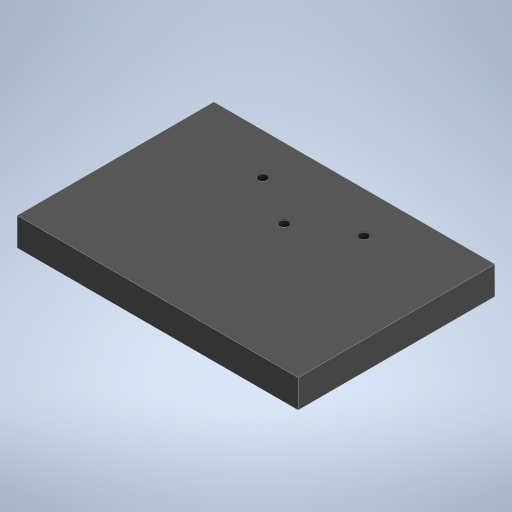
# Autodesk Inventor part: toe_sole_front
Saved by Autodesk Inventor 2024.1 (Build 281209000, 209)
## iProperties
Created: 2024-02-12
Part Number: toe_sole_front
Material: 一般
Document SubType Name: モデリング
Designer: hibik
Density: 1 g/cm^3
Appearance: 既定
Author: hibik
Autodesk Inventor part; units mm, degrees
ref_plane "YZ Plane" through (0, 0, 0) normal (1, 0, 0) x (0, 1, 0)
ref_plane "XZ Plane" through (0, 0, 0) normal (0, 1, 0) x (-1, 0, 0)
ref_plane "XY Plane" through (0, 0, 0) normal (0, 0, 1) x (1, 0, 0)
sketch "スケッチ1" plane through (0, 0, 0) normal (0, 1, 0) x (-1, 0, 0)
  line L0 (26, 0) -> (0, 0)
  line L1 (0, 0) -> (0, -15)
  line L2 (0, -15) -> (26, -15)
  line L3 (26, -15) -> (26, 0)
  line L4 (36.4849, 5.9511) -> (26, -20)
  line L5 (26, -20) -> (0, -20)
  line L6 (0, -20) -> (-10.4849, 5.9511)
  arc A0 (36.4849, 5.9511) -> (-10.4849, 5.9511) centre (13, -20) ccw
  line L7 (0, 0) -> (26, -15)
  line L8 (0, -15) -> (26, 0)
  line L9 (4, -2.3077) -> (22, -2.3077)
  line L10 (22, -2.3077) -> (22, -12.6923)
  line L11 (22, -12.6923) -> (4, -12.6923)
  line L12 (4, -12.6923) -> (4, -2.3077)
  circle A1 centre (4, -2.3077) radius 0.8
  circle A2 centre (4, -12.6923) radius 0.8
  circle A3 centre (22, -2.3077) radius 0.8
  circle A4 centre (22, -12.6923) radius 0.8
  circle A5 centre (13, -7.5) radius 0.8
  line L13 (38, 15) -> (-12, 15)
  line L14 (-12, 15) -> (-12, -20)
  line L15 (-12, -20) -> (38, -20)
  line L16 (38, -20) -> (38, 15)
  point P0 (22.6929, -13.0921)
  point P1 (21.2, -12.6923)
  point P2 (13, 15)
  point P3 (13, -7.5)
  point P4 (13, 15)
  point P5 (0, -20)
  dimension "d0" = 26
  dimension "d1" = 15
  dimension "d4" = 22
  dimension "d5" = 22
  dimension "d6" = 5
  dimension "d7" = 35
  dimension "d23" = 4
  dimension "d24" = 1.6
  dimension "d25" = 1.6
  dimension "d26" = 1.6
  dimension "d27" = 1.6
  dimension "d32" = 1.6
  dimension "d54" = 50
  dimension "d55" = 35
  constraints: 34 end point, 6 centre point, 6 coincident, 6 parallel, 5 point on line, 4 horizontal, 4 midpoint, 3 perpendicular, 2 point on circle, 1 collinear, 1 vertical alignment
  measures "d0" distance of L0.start L0.end
  measures "d1" distance of L2.end L0.start
  measures "d4" angle of L3 L4
  measures "d5" angle of L6 L1
  measures "d6" distance between parallel lines of L5 L2
  measures "d7" radius of A0
  measures "d23" distance between parallel lines of L1 L12
  measures "d24" diameter of A1
  measures "d25" diameter of A2
  measures "d26" diameter of A3
  measures "d27" diameter of A4
  measures "d32" diameter of A5
  measures "d54" distance of L13.start L13.end
  measures "d55" distance of L13.end L14.end
extrude "押し出し1" add sketch "スケッチ1" along normal blind 4 contours L8 A3 L9 A1 L7 L0 | L3 L7 A4 L10 A3 L8 | L7 A1 L12 A2 L8 L1 | L2 L8 A2 L11 A4 L7 | A3 L10 L8 | L8 L9 A3 | A1 L9 L7 | L7 L12 A1 | L10 A3 L8 | L8 A3 L9 | A3 L8 A5 L7 A1 L9 | L9 A1 L7 | L7 A1 L12 | A1 L7 A5 L8 A2 L12 | L11 A2 L8 A5 L7 A4 | A3 L10 A4 L7 A5 L8 | A0 L13 L16 L15 L4 | L4 L5 L6 A0 | A0 L6 L15 L14 L13
sketch "スケッチ5" plane through (0, 0, 0) normal (0, -1, 0) x (1, 0, 0)
  line L0 (12, -20) -> (-38, -20) projected
  line L1 (12, 15) -> (12, -20) projected
  line L2 (-38, 15) -> (12, 15) projected
  line L3 (-38, -20) -> (-38, 15) projected
  circle A0 centre (-13, -7.5) radius 0.8 projected
  circle A1 centre (-4, -12.6923) radius 0.8 projected
  circle A2 centre (-22, -12.6923) radius 0.8 projected
  circle A3 centre (-13, -7.5) radius 2.5
  circle A4 centre (-4, -12.6923) radius 2.5
  circle A5 centre (-22, -12.6923) radius 2.5
  line L4 (10, 12.5) -> (2, 12.5)
  line L5 (2, 12.5) -> (2, -17.5)
  line L6 (2, -17.5) -> (10, -17.5)
  line L7 (10, -17.5) -> (10, 12.5)
  line L8 (-28, 12.5) -> (-36, 12.5)
  line L9 (-36, 12.5) -> (-36, -17.5)
  line L10 (-36, -17.5) -> (-28, -17.5)
  line L11 (-28, -17.5) -> (-28, 12.5)
  point P0 (0, 0)
  point P1 (10, -2.5)
  point P2 (12, -2.5)
  point P3 (-28, -2.5)
  dimension "d56" = 5
  dimension "d57" = 5
  dimension "d58" = 5
  dimension "d61" = 8
  dimension "d62" = 30
  dimension "d63" = 2
  dimension "d64" = 2
  constraints: 16 end point, 4 parallel, 3 centre point, 3 coincident, 3 midpoint, 2 equal length, 2 horizontal, 2 horizontal alignment, 2 perpendicular
  measures "d56" diameter of A3
  measures "d57" diameter of A4
  measures "d58" diameter of A5
  measures "d61" distance of L6.end L5.end
  measures "d62" distance of L5.end L4.end
  measures "d63" distance between parallel lines of L1 L7
  measures "d64" distance between parallel lines of L3 L9
extrude "押し出し5" add sketch "スケッチ5" along normal blind 1 contours L0 L3 L2 L1
fillet "フィレット3" radius 1 8 edges at (6, -1, 12.5) (10, -1, -2.5) (6, -1, -17.5) (2, -1, -2.5) (-28, -1, -2.5) (-32, -1, -17.5) (-36, -1, -2.5) (-32, -1, 12.5)
equation "\"d5\" = d4"
equation "\"BendRadius\" = Thickness"
equation "\"BendReliefWidth\" = Thickness"
equation "\"BendReliefDepth\" = 0.5 * Thickness"
equation "\"CornerReliefSize\" = 4 * Thickness"
equation "\"MinimumRemnant\" = 2 * Thickness"
equation "\"TransitionRadius\" = BendRadius"
equation "\"JacobiRadiusSize\" = BendRadius"
equation "\"GapSize\" = Thickness"
equation "\"Thickness\" = 3.048"
